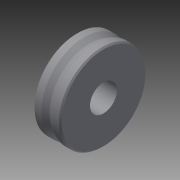
# Autodesk Inventor part: 625vv
Saved by Autodesk Inventor 2013 (Build 170138000, 138)
## iProperties
Created: 2014-05-21
Part Number: 625vv
Material: Generic
Document SubType Name: Modeling
Designer: employee
Density: 1 g/cm^3
Author: employee
Autodesk Inventor part; units mm, degrees
ref_plane "YZ Plane" through (0, 0, 0) normal (1, 0, 0) x (0, 1, 0)
ref_plane "XZ Plane" through (0, 0, 0) normal (0, 1, 0) x (-1, 0, 0)
ref_plane "XY Plane" through (0, 0, 0) normal (0, 0, 1) x (1, 0, 0)
sketch "Sketch1" plane through (0, 0, 0) normal (0, 0, 1) x (1, 0, 0)
  line L0 (-2.5, 2.5) -> (2.5, 2.5)
  line L1 (2.5, 2.5) -> (2.5, 8)
  line L2 (2.5, 8) -> (1, 8)
  line L3 (1, 8) -> (0, 7.5)
  line L4 (0, 7.5) -> (-1, 8)
  line L5 (-1, 8) -> (-2.5, 8)
  line L6 (-2.5, 8) -> (-2.5, 2.5)
  line L7 (-3.5, 0) -> (3.5, 0) projected
  point P0 (0, 0)
  point P1 (0, 2.5)
  dimension "d0" = 2.5
  dimension "d1" = 8
  dimension "d2" = 7.5
  dimension "d3" = 2
  dimension "d4" = 5
  constraints: 14 end point, 3 equal length, 2 parallel, 2 perpendicular, 1 horizontal, 1 midpoint, 1 vertical alignment
  measures "d0" distance from line of L0 point (0, 0)
  measures "d1" distance from line of L5 point (0, 0)
  measures "d2" distance of L3.end point (0, 0)
  measures "d3" distance of L2.end L4.end
  measures "d4" distance between parallel lines of L1 L6
revolve "Revolution1" add sketch "Sketch1" angle 360 about axis through (-10, 0, 0) along (1, 0, 0)
chamfer "Chamfer1" distance 0.25 angle 45 2 edges at (-2.5, -8, 0) (2.5, -8, 0)
body "Solid1"
